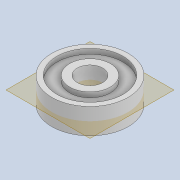
# Autodesk Inventor part: beraing_1_3_1
Saved by Autodesk Inventor 2020 (Build 240168000, 168)
## iProperties
Created: 2022-01-11
Part Number: beraing_1_3_1
Material: Generic
Document SubType Name: Modeling
Designer: Shuang Peng
Density: 1 g/cm^3
Appearance: Default
Author: Shuang Peng
Autodesk Inventor part; units mm, degrees
ref_plane "YZ Plane" through (0, 0, 0) normal (1, 0, 0) x (0, 1, 0)
ref_plane "XZ Plane" through (0, 0, 0) normal (0, 1, 0) x (-1, 0, 0)
ref_plane "XY Plane" through (0, 0, 0) normal (0, 0, 1) x (1, 0, 0)
sketch "Sketch1" plane through (0, 0, 0) normal (0, 1, 0) x (-1, 0, 0)
  circle A0 centre (0, 0) radius 0.5
  circle A1 centre (0, 0) radius 1.5
  dimension "d0" = 1
  dimension "d1" = 3
  constraints: 2 centre point, 2 coincident
  measures "d0" diameter of A0
  measures "d1" diameter of A1
extrude "Extrusion1" add sketch "Sketch1" along normal blind 1
sketch "Sketch2" plane through (0, 1, 0) normal (0, 1, 0) x (1, 0, 0)
  circle A0 centre (0, 0) radius 0.8
  circle A1 centre (0, 0) radius 1.3
  circle A2 centre (0, 0) radius 1.5 projected
  circle A3 centre (0, 0) radius 0.5 projected
  dimension "d4" = 0.3
  dimension "d5" = 0.2
  constraints: 2 centre point, 2 coincident
  measures "d4" radial gap between concentric circles of A0 A3
  measures "d5" radial gap between concentric circles of A2 A1
extrude "Extrusion2" cut sketch "Sketch2" against normal blind 0.2 contours A1
ref_plane "Work Plane1" through (0, 0.5, 0) normal (0, 1, 0) x (1, 0, 0)
mirror "Mirror1" about plane through (0, 0.5, 0) normal (0, 1, 0) of "Extrusion2"
body "Solid1"
